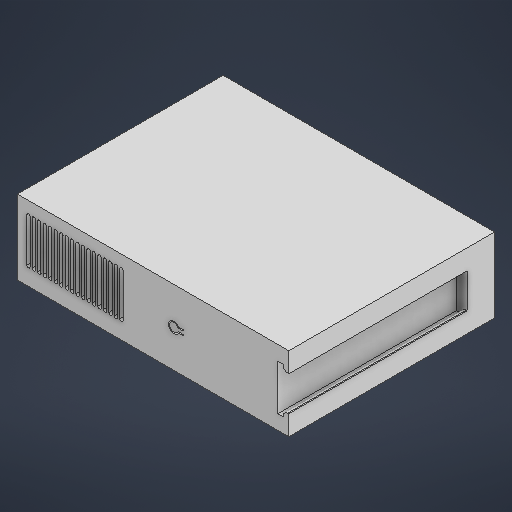
# Autodesk Inventor part: transmissor
Saved by Autodesk Inventor 2026.1 (Build 301233020, 233B)
## iProperties
Created: 2025-11-06
Part Number: transmissor
Material: Genérico
Document SubType Name: Modeling
Designer: luska
Density: 1 g/cm^3
Appearance: Padrão
Author: luska
## iProperties of the stored document transmissor_3DPrint.ipt
Created: 2025-11-11
Part Number: transmissor_3DPrint
Material: Genérico
Document SubType Name: Modeling
Designer: luska
Density: 1 g/cm^3
Appearance: Padrão
Author: luska
Autodesk Inventor part; units mm, degrees
ref_plane "YZ Plane" through (0, 0, 0) normal (1, 0, 0) x (0, 1, 0)
ref_plane "XZ Plane" through (0, 0, 0) normal (0, 1, 0) x (-1, 0, 0)
ref_plane "XY Plane" through (0, 0, 0) normal (0, 0, 1) x (1, 0, 0)
sketch "Esboço1" plane through (0, 0, 0) normal (0, 1, 0) x (-1, 0, 0)
  line L0 (100.4609, 54.9994) -> (-23.5391, 54.9994)
  line L1 (-23.5391, 54.9994) -> (-23.5391, -39.0006)
  line L2 (-23.5391, -39.0006) -> (100.4609, -39.0006)
  line L3 (100.4609, -39.0006) -> (100.4609, 54.9994)
  point P0 (0, 0)
  point P1 (-23.5391, 7.9994)
  point P2 (100.4609, 7.9994)
  dimension "d0" = 94
  dimension "d1" = 124
  constraints: 8 end point, 2 midpoint, 2 parallel, 1 horizontal, 1 perpendicular
  measures "d0" distance between parallel lines of L0 L2
  measures "d1" distance of point (-23.539, 7.999) point (100.461, 7.999)
extrude "Extrusão1" add sketch "Esboço1" along normal blind 34
sketch "Esboço2" plane through (0, 0, 0) normal (0, -1, 0) x (1, 0, 0)
  line L0 (16.5391, -37.0006) -> (-98.4609, -37.0006)
  line L1 (-98.4609, -37.0006) -> (-98.4609, 52.9994)
  line L2 (-98.4609, 52.9994) -> (16.5391, 52.9994)
  line L3 (16.5391, 52.9994) -> (16.5391, -37.0006)
  line L4 (23.5391, -39.0006) -> (-100.4609, -39.0006) projected
  line L5 (23.5391, 54.9994) -> (23.5391, -39.0006) projected
  line L6 (-100.4609, 54.9994) -> (23.5391, 54.9994) projected
  line L7 (-100.4609, -39.0006) -> (-100.4609, 54.9994) projected
  point P0 (0, 0)
  dimension "d4" = 2
  dimension "d5" = 7
  dimension "d6" = 2
  dimension "d7" = 2
  constraints: 8 end point, 2 parallel, 1 horizontal, 1 perpendicular
  measures "d4" distance between parallel lines of L4 L0
  measures "d5" distance between parallel lines of L5 L3
  measures "d6" distance between parallel lines of L6 L2
  measures "d7" distance between parallel lines of L7 L1
extrude "Extrusão2" cut sketch "Esboço2" against normal blind 32 contours L0 L1 L2 L3
sketch "Esboço3" plane through (0, 32, 0) normal (0, -1, 0) x (1, 0, 0)
  line L0 (16.5391, 52.9994) -> (16.5391, -37.0006) projected
  line L1 (-98.4609, -37.0006) -> (-98.4609, 52.9994) projected
  point P0 (0, 0)
sketch "Esboço4" plane through (0, 32, 0) normal (0, -1, 0) x (1, 0, 0)
  circle A0 centre (11.7391, -35.2006) radius 1.5
  circle A1 centre (10.8391, 41.5994) radius 1.5
  circle A2 centre (-16.2609, -32.3006) radius 1.5
  circle A3 centre (-47.0609, 41.2994) radius 1.5
  point P0 (0, 0)
  dimension "d11" = 3
  dimension "d15" = 3
  dimension "d16" = 3
  dimension "d17" = 3
  constraints: 4 centre point
  measures "d11" diameter of A0
  measures "d15" diameter of A1
  measures "d16" diameter of A2
  measures "d17" diameter of A3
extrude "Extrusão3" add sketch "Esboço4" along normal blind 5
sketch "Esboço5" plane through (-98.4609, 0, -37.0006) normal (0, 0, 1) x (1, 0, 0)
  point P0 (98.4609, 0)
sketch "Esboço7" plane through (23.5391, 0, 54.9994) normal (1, 0, 0) x (0, 0, -1)
  line L0 (81.52, 27.4) -> (0, 27.4)
  line L1 (0, 27.4) -> (0, 6.6)
  line L2 (0, 6.6) -> (81.52, 6.6)
  line L3 (81.52, 6.6) -> (81.52, 27.4)
  line L4 (0, 34) -> (94, 34) projected
  line L5 (0, 0) -> (94, 0) projected
  line L6 (0, 0) -> (0, 34) projected
  line L7 (94, 0) -> (94, 34) projected
  point P0 (54.9994, 0)
  point P1 (81.52, 17)
  dimension "d70" = 20.8
  dimension "d74" = 6.6
  dimension "d75" = 6.6
  dimension "d77" = 0
  dimension "d78" = 12.48
  constraints: 8 end point, 2 parallel, 1 horizontal, 1 midpoint, 1 perpendicular
  measures "d70" distance between parallel lines of L2 L0
  measures "d74" distance between parallel lines of L4 L0
  measures "d75" distance between parallel lines of L5 L2
  measures "d77" distance between parallel lines of L6 L1
  measures "d78" distance from line of L7 point (81.52, 17)
extrude "Extrusão5" cut sketch "Esboço7" against normal blind 5 contours L3 L2 L1 L0
sketch "Esboço10" plane through (23.5391, 0, -39.0006) normal (0, 0, -1) x (-1, 0, 0)
  point P0 (23.5391, 0)
sketch "Esboço12" plane through (23.5391, 27.4, -26.5206) normal (0, -1, 0) x (1, 0, 0)
  point P0 (-23.5391, 26.5206)
sketch "Esboço13" plane through (23.5391, 27.4, -26.5206) normal (0, -1, 0) x (1, 0, 0)
  line L0 (0, 81.52) -> (0, 0) projected
  line L1 (0, 0) -> (-5, 0) projected
  line L2 (0, 81.52) -> (-2.5, 81.52)
  line L3 (-2.5, 81.52) -> (-2.5, 0)
  line L4 (-2.5, 0) -> (0, 0)
  line L5 (0, 0) -> (0, 81.52)
  point P0 (-23.5391, 26.5206)
  dimension "d79" = 2.5
  constraints: 8 end point, 2 parallel, 1 horizontal, 1 midpoint, 1 perpendicular
  measures "d79" distance of L4.end L3.end
sketch "Esboço14" plane through (23.5391, 6.6, 54.9994) normal (0, 1, 0) x (1, 0, 0)
  line L0 (0, 81.52) -> (0, 0) projected
  line L1 (0, 81.52) -> (-5, 81.52) projected
  line L2 (0, 0) -> (-2.5, 0)
  line L3 (-2.5, 0) -> (-2.5, 81.52)
  line L4 (-2.5, 81.52) -> (0, 81.52)
  line L5 (0, 81.52) -> (0, 0)
  point P0 (-23.5391, 54.9994)
  dimension "d80" = 2.5
  constraints: 8 end point, 2 parallel, 1 horizontal, 1 midpoint, 1 perpendicular
  measures "d80" distance of L3.end L4.end
extrude "Extrusão8" add sketch "Esboço14" along normal blind 2.5
extrude "Extrusão9" add sketch "Esboço13" along normal blind 2.5
fillet "Arredondamento3" radius 2 2 edges at (21.0391, 24.9, 14.2394) (21.0391, 9.1, 14.2394)
sketch "Esboço15" plane through (23.5391, 0, -39.0006) normal (0, 0, -1) x (-1, 0, 0)
  circle A0 centre (30.8, 20.4) radius 3.25
  line L0 (0, 34) -> (124, 34) projected
  line L1 (0, 0) -> (0, 34) projected
  line L2 (47.2, 22.5) -> (39.2, 22.5)
  line L3 (39.2, 22.5) -> (39.2, 18.5)
  line L4 (39.2, 18.5) -> (47.2, 18.5)
  line L5 (47.2, 18.5) -> (47.2, 22.5)
  line L6 (115, 26) -> (95, 26)
  line L7 (95, 26) -> (95, 13)
  line L8 (95, 13) -> (115, 13)
  line L9 (115, 13) -> (115, 26)
  line L10 (124, 0) -> (124, 34) projected
  point P0 (23.5391, 0)
  dimension "d86" = 6.5
  dimension "d87" = 13.6
  dimension "d88" = 30.8
  dimension "d89" = 8
  dimension "d90" = 4
  dimension "d91" = 11.5
  dimension "d92" = 39.2
  dimension "d93" = 13
  dimension "d94" = 20
  dimension "d95" = 9
  dimension "d96" = 8
  constraints: 16 end point, 4 parallel, 2 horizontal, 2 perpendicular, 1 centre point
  measures "d86" diameter of A0
  measures "d87" distance from line of L0 A0.centre
  measures "d88" distance from line of L1 A0.centre
  measures "d89" distance of L4.end L3.end
  measures "d90" distance of L3.end L2.end
  measures "d91" distance between parallel lines of L0 L2
  measures "d92" distance between parallel lines of L1 L3
  measures "d93" distance between parallel lines of L8 L6
  measures "d94" distance between parallel lines of L7 L9
  measures "d95" distance between parallel lines of L10 L9
  measures "d96" distance between parallel lines of L0 L6
extrude "Extrusão10" cut sketch "Esboço15" against normal blind 2
sketch "Esboço16" plane through (23.5391, 0, -39.0006) normal (0, 0, -1) x (-1, 0, 0)
  point P0 (23.5391, 0)
sketch "Esboço17" plane through (0, 32, 0) normal (0, -1, 0) x (1, 0, 0)
  line L0 (-49.4609, 37.9994) -> (-50.4609, 37.9994)
  line L1 (-50.4609, 37.9994) -> (-50.4609, -37.0006)
  line L2 (-50.4609, -37.0006) -> (-49.4609, -37.0006)
  line L3 (-49.4609, -37.0006) -> (-49.4609, 37.9994)
  line L4 (16.5391, -37.0006) -> (-98.4609, -37.0006) projected
  line L5 (-98.4609, -37.0006) -> (-98.4609, 52.9994) projected
  line L6 (-50.4609, 37.9994) -> (-53.4609, 37.9994)
  line L7 (-53.4609, 37.9994) -> (-53.4609, 36.9994)
  line L8 (-53.4609, 36.9994) -> (-50.4609, 36.9994)
  line L9 (-50.4609, 36.9994) -> (-50.4609, 37.9994)
  point P0 (0, 0)
  point P1 (-49.9609, -37.0006)
  dimension "d99" = 1
  dimension "d100" = 75
  dimension "d101" = 0
  dimension "d102" = 48
  dimension "d103" = 3
  dimension "d104" = 1
  constraints: 16 end point, 4 parallel, 2 horizontal, 2 perpendicular, 1 midpoint
  measures "d99" distance of L2.end L1.end
  measures "d100" distance of L1.end L0.end
  measures "d101" distance from line of L4 point (-49.961, -37.001)
  measures "d102" distance between parallel lines of L5 L1
  measures "d103" distance of L8.end L7.end
  measures "d104" distance of L7.end L6.end
extrude "Extrusão11" add sketch "Esboço17" along normal blind 5
sketch "Esboço18" plane through (0, 0, 0) normal (0, -1, 0) x (1, 0, 0)
  point P0 (0, 0)
sketch "Esboço19" plane through (-47.0609, 27, 41.2994) normal (0, -1, 0) x (1, 0, 0)
  circle A0 centre (0, 0) radius 0.75
  circle A1 centre (57.9, 0.2909) radius 0.75
  circle A2 centre (57.9, 0.3) radius 1.5 projected
  point P0 (47.0609, -41.2994)
  dimension "d107" = 1.5
  dimension "d108" = 1.5
  dimension "d109" = 0
  constraints: 2 centre point
  measures "d107" diameter of A0
  measures "d108" diameter of A1
  measures "d109" horizontal distance of A2.centre A1.centre
extrude "Extrusão12" cut sketch "Esboço19" against normal blind 3 contours A0 | A1
sketch "Esboço20" plane through (11.7391, 27, -35.2006) normal (0, -1, 0) x (1, 0, 0)
  circle A0 centre (0, 0) radius 0.75
  circle A1 centre (-27.9901, 2.9) radius 0.75
  circle A2 centre (-28, 2.9) radius 1.5 projected
  point P0 (-11.7391, 35.2006)
  dimension "d112" = 1.5
  dimension "d113" = 1.5
  dimension "d114" = 0
  constraints: 2 centre point
  measures "d112" diameter of A0
  measures "d113" diameter of A1
  measures "d114" vertical distance of A2.centre A1.centre
extrude "Extrusão13" cut sketch "Esboço20" against normal blind 3 contours A0 | A1
sketch "Esboço21" plane through (-100.4609, 0, 54.9994) normal (0, 0, 1) x (1, 0, 0)
  arc A0 (73.7172, 18.155) -> (73.7172, 15.845) centre (71.5, 17) ccw
  line L0 (0, 0) -> (124, 0) projected
  line L1 (119, 6.6) -> (119, 27.4) projected
  arc A1 (73.3897, 17.655) -> (73.3897, 16.345) centre (71.5, 17) ccw
  line L2 (73.7172, 15.845) -> (75.7172, 15.845)
  line L3 (75.7172, 15.845) -> (75.7172, 16.345)
  line L4 (75.7172, 16.345) -> (73.3897, 16.345)
  line L5 (73.3897, 17.655) -> (75.7172, 17.655)
  line L6 (73.7172, 18.155) -> (75.7172, 18.155)
  line L7 (75.7172, 18.155) -> (75.7172, 17.655)
  point P0 (100.4609, 0)
  point P1 (119, 17)
  dimension "d117" = 5
  dimension "d118" = 17
  dimension "d119" = 47.5
  dimension "d120" = 4
  dimension "d121" = 2
  dimension "d122" = 0.5
  constraints: 12 end point, 4 point on circle, 3 perpendicular, 2 centre point, 2 horizontal, 1 coincident, 1 midpoint, 1 parallel, 1 point on line
  measures "d117" diameter of A0
  measures "d118" distance from line of L0 A0.centre
  measures "d119" distance of point (119, 17) A0.centre
  measures "d120" diameter of A1
  measures "d121" distance of L2.start L2.end
  measures "d122" distance of L2.end L3.end
extrude "Extrusão14" cut sketch "Esboço21" against normal blind 2
sketch "Esboço22" plane through (16.5391, 0, 52.9994) normal (0, 0, -1) x (-1, 0, 0)
  line L0 (42.5167, 13.9943) -> (42.5167, 19.9943)
  line L1 (42.5167, 19.9943) -> (48.5167, 19.9943)
  line L2 (48.5167, 19.9943) -> (48.5167, 13.9943)
  line L3 (0, 0) -> (0, 32) projected
  line L4 (48.8626, 20.4866) -> (42.1044, 20.4866)
  line L5 (42.1044, 20.4866) -> (42.1044, 13.5228)
  line L6 (48.8626, 13.5228) -> (48.8626, 20.4866)
  line L7 (42.5167, 13.9943) -> (42.5167, 13.5228)
  line L8 (48.5167, 13.9943) -> (48.5167, 13.5228)
  line L9 (42.1044, 13.5228) -> (42.5167, 13.5228)
  line L10 (48.5167, 13.5228) -> (48.8626, 13.5228)
  point P0 (16.5391, 0)
  constraints: 20 end point, 5 parallel, 3 perpendicular, 1 horizontal
extrude "Extrusão15" add sketch "Esboço22" along normal blind 5
sketch "Esboço23" plane through (16.5391, 0, 47.9994) normal (0, 0, -1) x (-1, 0, 0)
  line L0 (48.8626, 13.5228) -> (48.8626, 20.4866) projected
  line L1 (42.1044, 20.4866) -> (42.1044, 13.5228) projected
  line L2 (48.5167, 17.6588) -> (42.5139, 17.6588)
  line L3 (42.1044, 17.6588) -> (42.1044, 15.8583)
  line L4 (42.5167, 15.8583) -> (48.5167, 15.8583)
  line L5 (48.8626, 15.8583) -> (48.8626, 17.6588)
  line L6 (42.5167, 19.9943) -> (48.5167, 19.9943) projected
  line L7 (48.5167, 13.5228) -> (48.8626, 13.5228) projected
  line L8 (48.5167, 13.5228) -> (48.8626, 13.5228)
  line L9 (48.8626, 13.5228) -> (48.8626, 15.8583)
  line L10 (48.5167, 15.8583) -> (48.5167, 13.5228)
  line L11 (48.8626, 17.6588) -> (48.8626, 20.4866)
  line L12 (48.8626, 20.4866) -> (48.5167, 20.4866)
  line L13 (48.5167, 19.9943) -> (48.5167, 17.6588)
  line L14 (48.5167, 19.9943) -> (42.5139, 19.9943)
  line L15 (42.1044, 19.9943) -> (42.1044, 20.4866)
  line L16 (42.1044, 20.4866) -> (48.8626, 20.4866)
  line L17 (48.8626, 20.4866) -> (48.8626, 19.9943)
  line L18 (42.5167, 13.5228) -> (42.5167, 19.9943) projected
  line L19 (48.8626, 20.4866) -> (42.1044, 20.4866) projected
  line L20 (42.5167, 13.5228) -> (42.1044, 13.5228)
  line L21 (42.1044, 13.5228) -> (42.1044, 20.4866)
  line L22 (42.1044, 20.4866) -> (42.5167, 20.4866)
  line L23 (42.5139, 19.9943) -> (42.5139, 17.6588)
  line L24 (42.5167, 15.8583) -> (42.5167, 13.5228)
  line L25 (48.5167, 17.6588) -> (48.5167, 19.9943)
  line L26 (42.5139, 19.9943) -> (42.5139, 17.6588)
  line L27 (48.5167, 15.8583) -> (48.5167, 13.5228)
  point P0 (16.5391, 0)
  point P1 (48.6896, 13.5228)
  point P2 (42.5167, 15.8583)
  point P3 (42.5167, 17.6588)
  point P4 (44.8416, 19.9943)
  dimension "d131" = 2.3355
  dimension "d133" = 2.3355
  constraints: 44 end point, 10 parallel, 6 perpendicular, 4 horizontal, 3 point on line, 1 midpoint
  measures "d131" distance between parallel lines of L6 L2
  measures "d133" distance between parallel lines of L7 L4
extrude "Extrusão16" add sketch "Esboço23" along normal blind 1
sketch "Esboço24" plane through (-98.4609, 0, -37.0006) normal (0, 0, 1) x (1, 0, 0)
  line L0 (30, 3) -> (40, 3)
  line L1 (40, 3) -> (40, 5.5)
  line L2 (40, 5.5) -> (30, 5.5)
  line L3 (30, 5.5) -> (30, 3)
  line L4 (115, 0) -> (0, 0) projected
  line L5 (27, 13) -> (7, 13) projected
  line L6 (0, 0) -> (0, 32) projected
  line L7 (75, 3) -> (85, 3)
  line L8 (85, 3) -> (85, 5.5)
  line L9 (85, 5.5) -> (75, 5.5)
  line L10 (75, 5.5) -> (75, 3)
  line L11 (115, 0) -> (115, 32) projected
  point P0 (98.4609, 0)
  point P1 (75, 4.25)
  point P2 (40, 4.25)
  point P3 (85, 4.25)
  point P4 (80, 3)
  dimension "d136" = 10
  dimension "d139" = 2.5
  dimension "d140" = 3
  dimension "d141" = 7.5
  dimension "d142" = 30
  dimension "d143" = 10
  dimension "d144" = 2.5
  dimension "d147" = 30
  dimension "d148" = 3
  dimension "d149" = 35
  constraints: 16 end point, 4 midpoint, 4 parallel, 2 horizontal, 2 perpendicular
  measures "d136" distance of L2.end L1.end
  measures "d139" distance between parallel lines of L0 L2
  measures "d140" distance between parallel lines of L4 L0
  measures "d141" distance between parallel lines of L5 L2
  measures "d142" distance between parallel lines of L6 L3
  measures "d143" distance of L9.end L8.end
  measures "d144" distance of L8.end L7.end
  measures "d147" distance from line of L11 point (85, 4.25)
  measures "d148" distance from line of L4 point (80, 3)
  measures "d149" distance of point (75, 4.25) point (40, 4.25)
extrude "Extrusão17" cut sketch "Esboço24" against normal blind 1
sketch "Esboço25" plane through (16.5391, 0, 52.9994) normal (0, 0, -1) x (-1, 0, 0)
  line L0 (60, 4.078) -> (55, 4.078)
  line L1 (55, 4.078) -> (55, 1.578)
  line L2 (55, 1.578) -> (60, 1.578)
  line L3 (60, 1.578) -> (60, 4.078)
  line L4 (0, 0) -> (0, 32) projected
  point P0 (16.5391, 0)
  point P1 (60, 2.828)
  point P2 (55, 2.828)
  dimension "d152" = 2.5
  dimension "d153" = 5
  dimension "d154" = 55
  constraints: 8 end point, 2 midpoint, 2 parallel, 1 horizontal, 1 perpendicular
  measures "d152" distance between parallel lines of L2 L0
  measures "d153" distance from line of point (60, 2.828) L1
  measures "d154" distance from line of L4 point (55, 2.828)
extrude "Extrusão18" add sketch "Esboço25" along normal blind 3
sketch "Esboço26" plane through (-43.4609, 1.578, 52.9994) normal (0, -1, 0) x (1, 0, 0)
  circle A0 centre (2.5, -1.5) radius 0.75
  line L0 (5, -3) -> (0, -3) projected
  line L1 (0, 0) -> (0, -3) projected
  point P0 (43.4609, -52.9994)
  dimension "d157" = 1.5
  dimension "d158" = 1.5
  dimension "d159" = 2.5
  constraints: 1 centre point
  measures "d157" diameter of A0
  measures "d158" distance from line of L0 A0.centre
  measures "d159" distance from line of L1 A0.centre
extrude "Extrusão19" cut sketch "Esboço26" against normal blind 3
sketch "Esboço27" plane through (-100.4609, 0, 54.9994) normal (0, 0, 1) x (1, 0, 0)
  line L0 (47.5, 28) -> (47.5, 8) construction
  line L1 (46.75, 28) -> (46.75, 8)
  line L2 (48.25, 8) -> (48.25, 28)
  arc A0 (48.25, 28) -> (46.75, 28) centre (47.5, 28) ccw
  arc A1 (46.75, 8) -> (48.25, 8) centre (47.5, 8) ccw
  line L3 (0, 34) -> (124, 34) projected
  line L4 (119, 6.6) -> (119, 27.4) projected
  line L5 (47.5, 18) -> (46.75, 18)
  line L6 (45, 28) -> (45, 8) construction
  line L7 (44.25, 28) -> (44.25, 8)
  line L8 (45.75, 8) -> (45.75, 28)
  arc A2 (45.75, 28) -> (44.25, 28) centre (45, 28) ccw
  arc A3 (44.25, 8) -> (45.75, 8) centre (45, 8) ccw
  line L9 (42.5, 28) -> (42.5, 8) construction
  line L10 (41.75, 28) -> (41.75, 8)
  line L11 (43.25, 8) -> (43.25, 28)
  arc A4 (43.25, 28) -> (41.75, 28) centre (42.5, 28) ccw
  arc A5 (41.75, 8) -> (43.25, 8) centre (42.5, 8) ccw
  line L12 (40, 28) -> (40, 8) construction
  line L13 (39.25, 28) -> (39.25, 8)
  line L14 (40.75, 8) -> (40.75, 28)
  arc A6 (40.75, 28) -> (39.25, 28) centre (40, 28) ccw
  arc A7 (39.25, 8) -> (40.75, 8) centre (40, 8) ccw
  line L15 (37.5, 28) -> (37.5, 8) construction
  line L16 (36.75, 28) -> (36.75, 8)
  line L17 (38.25, 8) -> (38.25, 28)
  arc A8 (38.25, 28) -> (36.75, 28) centre (37.5, 28) ccw
  arc A9 (36.75, 8) -> (38.25, 8) centre (37.5, 8) ccw
  line L18 (35, 28) -> (35, 8) construction
  line L19 (34.25, 28) -> (34.25, 8)
  line L20 (35.75, 8) -> (35.75, 28)
  arc A10 (35.75, 28) -> (34.25, 28) centre (35, 28) ccw
  arc A11 (34.25, 8) -> (35.75, 8) centre (35, 8) ccw
  line L21 (32.5, 28) -> (32.5, 8) construction
  line L22 (31.75, 28) -> (31.75, 8)
  line L23 (33.25, 8) -> (33.25, 28)
  arc A12 (33.25, 28) -> (31.75, 28) centre (32.5, 28) ccw
  arc A13 (31.75, 8) -> (33.25, 8) centre (32.5, 8) ccw
  line L24 (30, 28) -> (30, 8) construction
  line L25 (29.25, 28) -> (29.25, 8)
  line L26 (30.75, 8) -> (30.75, 28)
  arc A14 (30.75, 28) -> (29.25, 28) centre (30, 28) ccw
  arc A15 (29.25, 8) -> (30.75, 8) centre (30, 8) ccw
  line L27 (27.5, 28) -> (27.5, 8) construction
  line L28 (26.75, 28) -> (26.75, 8)
  line L29 (28.25, 8) -> (28.25, 28)
  arc A16 (28.25, 28) -> (26.75, 28) centre (27.5, 28) ccw
  arc A17 (26.75, 8) -> (28.25, 8) centre (27.5, 8) ccw
  line L30 (25, 28) -> (25, 8) construction
  line L31 (24.25, 28) -> (24.25, 8)
  line L32 (25.75, 8) -> (25.75, 28)
  arc A18 (25.75, 28) -> (24.25, 28) centre (25, 28) ccw
  arc A19 (24.25, 8) -> (25.75, 8) centre (25, 8) ccw
  line L33 (22.5, 28) -> (22.5, 8) construction
  line L34 (21.75, 28) -> (21.75, 8)
  line L35 (23.25, 8) -> (23.25, 28)
  arc A20 (23.25, 28) -> (21.75, 28) centre (22.5, 28) ccw
  arc A21 (21.75, 8) -> (23.25, 8) centre (22.5, 8) ccw
  line L36 (20, 28) -> (20, 8) construction
  line L37 (19.25, 28) -> (19.25, 8)
  line L38 (20.75, 8) -> (20.75, 28)
  arc A22 (20.75, 28) -> (19.25, 28) centre (20, 28) ccw
  arc A23 (19.25, 8) -> (20.75, 8) centre (20, 8) ccw
  line L39 (17.5, 28) -> (17.5, 8) construction
  line L40 (16.75, 28) -> (16.75, 8)
  line L41 (18.25, 8) -> (18.25, 28)
  arc A24 (18.25, 28) -> (16.75, 28) centre (17.5, 28) ccw
  arc A25 (16.75, 8) -> (18.25, 8) centre (17.5, 8) ccw
  line L42 (15, 28) -> (15, 8) construction
  line L43 (14.25, 28) -> (14.25, 8)
  line L44 (15.75, 8) -> (15.75, 28)
  arc A26 (15.75, 28) -> (14.25, 28) centre (15, 28) ccw
  arc A27 (14.25, 8) -> (15.75, 8) centre (15, 8) ccw
  line L45 (0, 0) -> (0, 34) projected
  line L46 (13.25, 8) -> (13.25, 28)
  line L47 (12.5, 28) -> (12.5, 8) construction
  line L48 (11.75, 28) -> (11.75, 8)
  arc A28 (13.25, 28) -> (11.75, 28) centre (12.5, 28) ccw
  arc A29 (11.75, 8) -> (13.25, 8) centre (12.5, 8) ccw
  arc A30 (14.25, 8) -> (15.75, 8) centre (15, 8) ccw
  line L49 (10.75, 8) -> (10.75, 28)
  line L50 (10, 28) -> (10, 8) construction
  line L51 (9.25, 28) -> (9.25, 8)
  arc A31 (10.75, 28) -> (9.25, 28) centre (10, 28) ccw
  arc A32 (9.25, 8) -> (10.75, 8) centre (10, 8) ccw
  arc A33 (11.75, 8) -> (13.25, 8) centre (12.5, 8) ccw
  line L52 (8.25, 8) -> (8.25, 28)
  line L53 (7.5, 28) -> (7.5, 8) construction
  line L54 (6.75, 28) -> (6.75, 8)
  arc A34 (8.25, 28) -> (6.75, 28) centre (7.5, 28) ccw
  arc A35 (6.75, 8) -> (8.25, 8) centre (7.5, 8) ccw
  arc A36 (9.25, 8) -> (10.75, 8) centre (10, 8) ccw
  line L55 (5.75, 8) -> (5.75, 28)
  line L56 (5, 28) -> (5, 8) construction
  line L57 (4.25, 28) -> (4.25, 8)
  arc A37 (5.75, 28) -> (4.25, 28) centre (5, 28) ccw
  arc A38 (4.25, 8) -> (5.75, 8) centre (5, 8) ccw
  arc A39 (6.75, 8) -> (8.25, 8) centre (7.5, 8) ccw
  point P0 (100.4609, 0)
  point P1 (45, 18)
  point P2 (42.5, 18)
  point P3 (40, 18)
  point P4 (37.5, 18)
  point P5 (35, 18)
  point P6 (32.5, 18)
  point P7 (30, 18)
  point P8 (27.5, 18)
  point P9 (25, 18)
  point P10 (22.5, 18)
  point P11 (20, 18)
  point P12 (17.5, 18)
  point P13 (15, 18)
  point P14 (12.5, 18)
  point P15 (10, 18)
  point P16 (7.5, 18)
  point P17 (5, 18)
  dimension "d162" = 20
  dimension "d163" = 1.5
  dimension "d164" = 6
  dimension "d168" = 2.5
  dimension "d173" = 15
  dimension "d176" = 2.5
  constraints: 146 end point, 80 point on circle, 40 centre point, 4 tangent, 3 horizontal, 2 midpoint, 1 parallel, 1 vertical, 220 other
  measures "d162" distance of L0.start L0.end
  measures "d163" diameter of A1
  measures "d164" distance from line of L3 L0.start
  measures "d168" distance of L1.start L7.start
  measures "d173" distance between parallel lines of L45 L42
  measures "d176" distance of L44.start L46.start
extrude "Extrusão20" cut sketch "Esboço27" against normal blind 3
